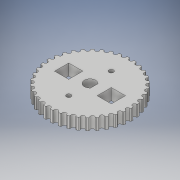
# Autodesk Inventor part: nhk27
Saved by Autodesk Inventor 2019 (Build 230136000, 136)
## iProperties
Created: 2022-02-27
Part Number: nhk27
Material: 一般
Document SubType Name: Sheet Metal
Designer: yuta
Density: 1 g/cm^3
Sheet Metal Rule: Default_mm
Appearance: 既定
Author: yuta
Autodesk Inventor part; units mm, degrees
ref_plane "YZ Plane" through (0, 0, 0) normal (1, 0, 0) x (0, 1, 0)
ref_plane "XZ Plane" through (0, 0, 0) normal (0, 1, 0) x (-1, 0, 0)
ref_plane "XY Plane" through (0, 0, 0) normal (0, 0, 1) x (1, 0, 0)
sketch "スケッチ1" plane through (0, 0, 0) normal (0, 1, 0) x (-1, 0, 0)
  circle A0 centre (0, 0) radius 30.24 construction
  arc A1 (2.9866, -29.5193) -> (1.262, -29.6431) centre (0, 0) ccw construction
  circle A2 centre (0, 0) radius 27.74 construction
  arc A3 (1.37, -29.1022) -> (0, -27.74) centre (0, -29.11) ccw
  arc A4 (4.5659, -27.3617) -> (3.4388, -28.9308) centre (4.7913, -28.713) ccw
  arc A5 (1.37, -29.1022) -> (1.9128, -29.6083) centre (1.88, -29.0993) ccw
  arc A6 (2.9866, -29.5193) -> (3.4388, -28.9308) centre (2.9353, -29.0119) ccw
  line L0 (4.5659, -27.3617) -> (0, 0)
  line L1 (0, 0) -> (0, -27.74)
  arc A7 (1.9128, -29.6083) -> (2.9866, -29.5193) centre (0, 0) ccw construction
  arc A8 (1.262, -29.6431) -> (1.9128, -29.6083) centre (0, 0) ccw construction
  arc A9 (1.8937, -29.6092) -> (2.9866, -29.5193) centre (1.2253, -14.7868) ccw
  dimension "d0" = 60.48
  dimension "d1" = 59.34
  dimension "d3" = 55.48
  dimension "d4" = 2.74
  dimension "d5" = 2.74
  dimension "d6" = 0.57
  dimension "d7" = 1.93
  dimension "d8" = 1.02
  dimension "d9" = 1.02
  dimension "d10" = 9.474
  constraints: 21 point on circle, 10 centre point, 6 tangent, 4 end point, 2 coincident, 1 vertical
  measures "d0" diameter of A0
  measures "d1" diameter of A1
  measures "d3" diameter of A2
  measures "d4" diameter of A3
  measures "d5" diameter of A4
  measures "d6" radial gap between concentric circles of A1 A0
  measures "d7" radial gap between concentric circles of A2 A1
  measures "d8" diameter of A5
  measures "d9" diameter of A6
  measures "d10" angle of L1 L0
extrude "押し出し1" add sketch "スケッチ1" along normal blind 8
pattern_circular "円形状パターン1" count 38 over 360 about axis through (0, 0, 0) along (0, 1, 0) of "押し出し1"
sketch "スケッチ2" plane through (0, 8, 0) normal (0, 1, 0) x (1, 0, 0)
  circle A0 centre (0, 0) radius 4
  line L0 (3, -2.6458) -> (3, 2.6458)
  point P0 (3, 0)
  dimension "d16" = 8
  dimension "d17" = 3
  constraints: 2 end point, 2 point on circle, 1 centre point, 1 coincident, 1 vertical
  measures "d16" diameter of A0
  measures "d17" distance of A0.centre point (3, 0)
extrude "押し出し2" cut sketch "スケッチ2" against normal blind 8 contours L0 A0 picked at (-0.1458, -1.2472)
sketch "スケッチ3" plane through (0, 8, 0) normal (0, 1, 0) x (1, 0, 0)
  line L0 (-20, -5) -> (-10, -5)
  line L1 (-10, -5) -> (-10, 5)
  line L2 (-10, 5) -> (-20, 5)
  line L3 (-20, 5) -> (-20, -5)
  line L4 (10, -5) -> (20, -5)
  line L5 (20, -5) -> (20, 5)
  line L6 (20, 5) -> (10, 5)
  line L7 (10, 5) -> (10, -5)
  point P0 (0, 0)
  dimension "d20" = 10
  dimension "d21" = 10
  dimension "d22" = 10
  dimension "d23" = 10
  dimension "d24" = 5
  dimension "d25" = 20
  dimension "d26" = 20
  constraints: 16 end point, 4 parallel, 2 horizontal, 2 perpendicular, 1 point on line
  measures "d20" distance of L2.end L1.end
  measures "d21" distance of L1.end L0.end
  measures "d22" distance of L6.end L5.end
  measures "d23" distance of L5.end L4.end
  measures "d24" distance from line of point (0, 0) L0
  measures "d25" distance from line of point (0, 0) L3
  measures "d26" distance from line of point (0, 0) L5
extrude "押し出し3" cut sketch "スケッチ3" against normal blind 8
sketch "スケッチ4" plane through (0, 8, 0) normal (0, 1, 0) x (1, 0, 0)
  circle A0 centre (0, 15) radius 1.6
  circle A1 centre (0, -15) radius 1.6
  point P0 (0, 0)
  dimension "d29" = 3.2
  dimension "d30" = 3.2
  dimension "d31" = 15
  dimension "d32" = 15
  constraints: 2 centre point
  measures "d29" diameter of A0
  measures "d30" diameter of A1
  measures "d31" distance of A0.centre point (0, 0)
  measures "d32" distance of A1.centre point (0, 0)
hole "穴1" at (0, 8, 15) at (0, 8, -15) direction (0, -1, 0) diameter 3.2 depth 8
equation "\"BendRadius\" = Thickness"
equation "\"BendReliefWidth\" = Thickness"
equation "\"BendReliefDepth\" = 0.5 * Thickness"
equation "\"CornerReliefSize\" = 4 * Thickness"
equation "\"MinimumRemnant\" = 2 * Thickness"
equation "\"TransitionRadius\" = BendRadius"
equation "\"JacobiRadiusSize\" = BendRadius"
equation "\"GapSize\" = Thickness"
equation "\"Thickness\" = 0.5"
